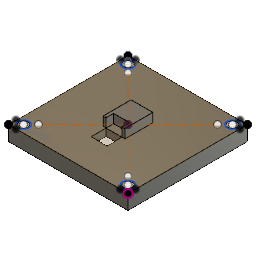
Top Part Enclosure (Autodesk Fusion 360 design; units mm, degrees)
Autodesk Fusion 360 part; units mm, degrees
sketch "Sketch1" plane through (0, 0, 0) normal (0, 1, 0) x (1, 0, 0)
  line L0 (40, -40) -> (-40, -40)
  line L1 (-40, -40) -> (-40, 40)
  line L2 (-40, 40) -> (40, 40)
  line L3 (40, 40) -> (40, -40)
  line L4 (40, -40) -> (-40, 40) construction
  line L5 (-40, -40) -> (40, 40) construction
  dimension "d1" = 80
  dimension "d2" = 80
extrude "Extrude1" add sketch "Sketch1" along normal blind 50
sketch "Sketch2" plane through (0, 50, 0) normal (0, 1, 0) x (-1, 0, 0)
  line L0 (-40, -40) -> (40, -40)
  line L1 (40, -40) -> (40, 40)
  line L2 (40, 40) -> (-40, 40)
  line L3 (-40, 40) -> (-40, -40)
  line L4 (7.3005, -9.361) -> (-7.3005, -9.361)
  line L5 (-7.3005, -9.361) -> (-7.3005, 9.361)
  line L6 (-7.3005, 9.361) -> (7.3005, 9.361)
  line L7 (7.3005, 9.361) -> (7.3005, -9.361)
  line L8 (7.3005, -9.361) -> (-7.3005, 9.361) construction
  line L9 (-7.3005, -9.361) -> (7.3005, 9.361) construction
  dimension "d5" = 14.601
  dimension "d6" = 18.722
extrude "Extrude2" add sketch "Sketch2" along normal blind 6 contours L4 L5 L6 L7
sketch "Sketch3" plane through (0, 0, 9.361) normal (0, 0, 1) x (1, 0, 0)
  line L0 (-7.3005, 50) -> (7.3005, 50)
  line L1 (7.3005, 50) -> (7.3005, 56)
  line L2 (7.3005, 56) -> (-7.3005, 56)
  line L3 (-7.3005, 56) -> (-7.3005, 50)
  line L4 (-7.3005, 50) -> (-5.3005, 50)
  line L5 (7.3005, 50) -> (5.3005, 50)
  line L6 (-5.3005, 50) -> (-5.3005, 54.5)
  line L7 (5.3005, 50) -> (-5.3005, 50)
  line L8 (-5.3005, 50) -> (-5.3005, 54.5)
  line L9 (-5.3005, 54.5) -> (5.3005, 54.5)
  line L10 (5.3005, 54.5) -> (5.3005, 50)
  dimension "d9" = 2
  dimension "d10" = 2
  dimension "d11" = 4.5
extrude "Extrude3" cut sketch "Sketch3" against normal blind 5 contours L0 L6 L7 L8 L9 L10
sketch "Sketch4" plane through (0, 56, 0) normal (0, 1, 0) x (-1, 0, 0)
  line L0 (7.3005, 9.361) -> (-7.3005, 9.361)
  line L1 (-7.3005, 9.361) -> (-7.3005, -9.361)
  line L2 (-7.3005, -9.361) -> (7.3005, -9.361)
  line L3 (7.3005, -9.361) -> (7.3005, 9.361)
  line L4 (7.3005, 9.361) -> (5.3005, 9.361)
  line L5 (-7.3005, 9.361) -> (-5.3005, 9.361)
  line L6 (5.3005, 9.361) -> (5.3005, 4.361)
  line L7 (5.3005, 9.361) -> (5.3005, 6.861)
  line L8 (-5.3005, 9.361) -> (5.3005, 9.361)
  line L9 (5.3005, 9.361) -> (5.3005, 4.361)
  line L10 (5.3005, 4.361) -> (-5.3005, 4.361)
  line L11 (-5.3005, 4.361) -> (-5.3005, 9.361)
extrude "Extrude4" cut sketch "Sketch4" against normal blind 2 contours L0 L6 L7 L8 L9 L10 L11
sketch "Sketch5" plane through (0, 50, 0) normal (0, 1, 0) x (-1, 0, 0)
  line L0 (7.3005, 9.361) -> (7.3005, -9.361)
  line L1 (7.3005, -9.361) -> (-7.3005, -9.361)
  line L2 (-7.3005, -9.361) -> (-7.3005, 9.361)
  line L3 (-7.3005, 9.361) -> (-5.3005, 9.361)
  line L4 (-5.3005, 9.361) -> (-5.3005, 4.361)
  line L5 (-5.3005, 4.361) -> (5.3005, 4.361)
  line L6 (5.3005, 4.361) -> (5.3005, 9.361)
  line L7 (5.3005, 9.361) -> (7.3005, 9.361)
  line L8 (-40, -40) -> (40, -40)
  line L9 (40, -40) -> (40, 40)
  line L10 (40, 40) -> (-40, 40)
  line L11 (-40, 40) -> (-40, -40)
  line L12 (5.3005, 9.361) -> (5.3005, 19.361)
  line L13 (-5.3005, 9.361) -> (-5.3005, 19.361)
  line L14 (5.3005, 9.361) -> (-5.3005, 9.361)
  line L15 (-5.3005, 9.361) -> (-5.3005, 19.361)
  line L16 (-5.3005, 19.361) -> (5.3005, 19.361)
  line L17 (5.3005, 19.361) -> (5.3005, 9.361)
  dimension "d16" = 10
  dimension "d17" = 10
extrude "Extrude5" cut sketch "Sketch5" against normal up to surface (50 mm away) contours L12 L13 L14 L15 L16 L17
sketch "Sketch6" plane through (0, 0, 40) normal (0, 0, 1) x (1, 0, 0)
  line L0 (-40, 0) -> (40, 0)
  line L1 (40, 50) -> (-40, 50)
  line L2 (-40, 50) -> (-40, 0)
sketch "Sketch7" plane through (0, 50, 0) normal (0, 1, 0) x (-1, 0, 0)
  line L0 (-40, -40) -> (40, -40)
  line L1 (40, -40) -> (40, 40)
  line L2 (40, 40) -> (-40, 40)
  line L3 (-40, 40) -> (-40, -40)
  line L4 (-5.3005, 9.361) -> (-5.3005, 19.361)
  line L5 (-5.3005, 19.361) -> (5.3005, 19.361)
  line L6 (5.3005, 19.361) -> (5.3005, 9.361)
  line L7 (5.3005, 9.361) -> (7.3005, 9.361)
  line L8 (7.3005, 9.361) -> (7.3005, -9.361)
  line L9 (7.3005, -9.361) -> (-7.3005, -9.361)
  line L10 (-7.3005, -9.361) -> (-7.3005, 9.361)
  line L11 (-7.3005, 9.361) -> (-5.3005, 9.361)
  line L12 (40, -40) -> (35, -40)
  line L13 (-40, -40) -> (-35, -40)
  line L14 (40, 40) -> (35, 40)
  line L15 (-40, 40) -> (-35, 40)
  line L16 (40, -40) -> (40, -35)
  line L17 (-40, -40) -> (-40, -35)
  line L18 (40, 40) -> (40, 35)
  line L19 (-40, 40) -> (-40, 35)
  circle A0 centre (35, -35) radius 3.75
  circle A1 centre (35, 35) radius 3.75
  circle A2 centre (-35, -35) radius 3.75
  circle A3 centre (-35, 35) radius 3.75
  line L20 (-30, -30) -> (30, 30) construction
  line L21 (30, -30) -> (-30, 30) construction
  dimension "d20" = 5
  dimension "d21" = 5
  dimension "d22" = 5
  dimension "d23" = 5
  dimension "d24" = 5
  dimension "d25" = 5
  dimension "d26" = 5
  dimension "d27" = 5
  dimension "d28" = 7.5
  dimension "d29" = 7.5
  dimension "d30" = 7.5
  dimension "d31" = 7.5
  dimension "d41" = 60
  dimension "d42" = 60
  measures "d28" diameter of A0
  measures "d29" diameter of A1
  measures "d30" diameter of A2
  measures "d31" diameter of A3
move_face "OffsetFaces2" offset -40 1 faces at (-1.7668, 0, -23.5463)
extrude "Extrude10" cut sketch "Sketch7" against normal blind 10 contours A0
extrude "Extrude11" cut sketch "Sketch7" against normal blind 10 contours A2
extrude "Extrude12" cut sketch "Sketch7" against normal blind 10 contours A1
extrude "Extrude13" cut sketch "Sketch7" against normal blind 10 contours A3
thread "Thread5" "ISO Metric profile 7.0 M7x1 6H" major diameter 7.1472 minor diameter 6.0355 pitch 1 angle 60 resizes the face on face at (-38.7453, 43.3333, -35.1869)
thread "Thread6" "ISO Metric profile 7.0 M7x1 6H" major diameter 7.1472 minor diameter 6.0355 pitch 1 angle 60 resizes the face on face at (-38.7453, 43.3333, 34.8131)
thread "Thread7" "ISO Metric profile 7.0 M7x1 6H" major diameter 7.1472 minor diameter 6.0355 pitch 1 angle 60 resizes the face on face at (31.2547, 43.3333, 34.8131)
thread "Thread8" "ISO Metric profile 7.0 M7x1 6H" major diameter 7.1472 minor diameter 6.0355 pitch 1 angle 60 resizes the face on face at (31.2547, 43.3333, -35.1869)
sketch "Sketch8" plane through (0, 40, 0) normal (0, -1, 0) x (1, 0, 0)
  circle A0 centre (35, 35) radius 3.0178
  circle A1 centre (-35, 35) radius 3.0178
  circle A2 centre (35, -35) radius 3.0178
  circle A3 centre (-35, -35) radius 3.0178
  line L0 (-5.3005, 9.361) -> (-5.3005, 19.361)
  line L1 (-5.3005, 19.361) -> (5.3005, 19.361)
  line L2 (5.3005, 19.361) -> (5.3005, 9.361)
  line L3 (5.3005, 9.361) -> (-5.3005, 9.361)
  line L4 (-40, -40) -> (40, -40)
  line L5 (40, -40) -> (40, 40)
  line L6 (40, 40) -> (-40, 40)
  line L7 (-40, 40) -> (-40, -40)
  line L8 (30, -30) -> (-30, -30)
  line L9 (-30, -30) -> (-30, 30)
  line L10 (-30, 30) -> (30, 30)
  line L11 (30, 30) -> (30, -30)
  line L12 (30, -30) -> (-30, 30) construction
  line L13 (-30, -30) -> (30, 30) construction
  dimension "d52" = 60
  dimension "d53" = 60
extrude "Extrude14" cut sketch "Sketch8" against normal blind 5 contours L8 L9 L10 L11
extrude "Extrude6" [suppressed]
extrude "Extrude7" [suppressed]
extrude "Extrude8" [suppressed]
extrude "Extrude9" [suppressed]
thread "Thread1" [suppressed]
thread "Thread2" [suppressed]
thread "Thread3" [suppressed]
thread "Thread4" [suppressed]
move_face "OffsetFaces1" [suppressed]
